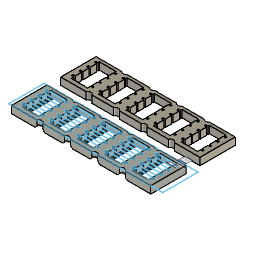
2025_11_30_Stock20Pico2W v6 (Autodesk Fusion 360 design; units mm, degrees)
Autodesk Fusion 360 part; units mm, degrees
note: some values were not read from the file. Set by a fixed rule: which face or edge a step refers to.
sketch "Sketch1" plane through (0, 0, 0) normal (0, 0, 1) x (1, 0, 0)
  line L0 (71.5, 36) -> (-71.5, 36)
  line L1 (-71.5, 36) -> (-71.5, -36)
  line L2 (-71.5, -36) -> (71.5, -36)
  line L3 (71.5, -36) -> (71.5, 36)
  line L4 (71.5, 36) -> (-71.5, -36) construction
  line L5 (-71.5, 36) -> (71.5, -36) construction
  line L6 (71.5, -36) -> (96.5, -36)
  line L7 (96.5, -36) -> (96.5, -14)
  line L8 (96.5, -14) -> (71.5, -14)
  line L9 (71.5, -14) -> (71.5, -36)
  line L10 (71.5, 36) -> (96.5, 36)
  line L11 (96.5, 36) -> (96.5, 14)
  line L12 (96.5, 14) -> (71.5, 14)
  line L13 (71.5, 14) -> (71.5, 36)
  line L14 (71.5, 14) -> (96.5, 14)
  line L15 (96.5, 14) -> (96.5, -14)
  line L16 (96.5, -14) -> (71.5, -14)
  line L17 (71.5, -14) -> (71.5, 14)
  dimension "d1" = 143
  dimension "d2" = 72
  dimension "d5" = 25
  dimension "d6" = 22
  dimension "d7" = 22
  constraint horizontal L0
  constraint perpendicular L0 L1
  constraint parallel L0 L2
  constraint parallel L1 L3
  constraint coincident L4 origin
  constraint coincident L5 origin
  constraint horizontal L6
  constraint vertical L7
  constraint horizontal L8
  constraint vertical L9
  constraint horizontal L10
  constraint vertical L11
  constraint horizontal L12
  constraint vertical L13
  constraint horizontal L14
  constraint vertical L15
  constraint horizontal L16
  constraint vertical L17
  measures "d1" distance of L1.end L2.end
  measures "d2" distance of L0.end L1.end
  measures "d5" distance of L2.end L6.end
  measures "d6" distance of L2.end L8.end
  measures "d7" distance of L0.start L12.end
extrude "Extrude1" add sketch "Sketch1" along normal blind 65 contours L0 L1 L2 L3 L9 L13 L17 makes body 1
sketch "Sketch2" plane through (0, 0, 0) normal (0, 0, 1) x (1, 0, 0)
  line L0 (67.3908, -47.7259) -> (44.3908, -47.7259)
  line L1 (44.3908, -47.7259) -> (44.3908, -49.2259)
  line L2 (44.3908, -49.2259) -> (67.3908, -49.2259)
  line L3 (67.3908, -49.2259) -> (67.3908, -47.7259)
  line L4 (64.8908, -52.2259) -> (46.8908, -52.2259)
  line L5 (46.8908, -52.2259) -> (46.8908, -47.7259)
  line L6 (64.8908, -47.7259) -> (64.8908, -52.2259)
  line L7 (64.8908, -52.2259) -> (51.3908, -47.7259) construction
  line L8 (46.8908, -52.2259) -> (60.3908, -47.7259) construction
  point P0 (55.8908, -49.2259)
  dimension "d8" = 23
  dimension "d9" = 1.5
  constraint horizontal L0
  constraint vertical L1
  constraint horizontal L2
  constraint vertical L3
  constraint horizontal L4
  constraint perpendicular L4 L5
  constraint parallel L5 L6
  constraint coincident L7 P0
  constraint coincident L8 P0
  constraint midpoint L2 P0
  constraint coincident L0 L6.start
  constraint coincident L0 L5.end
  constraint coincident L0 L7.end
  constraint coincident L0 L8.end
  measures "d8" distance of L0.start L0.end
  measures "d9" distance of L0.start L2.end
extrude "Extrude2" add sketch "Sketch2" along normal blind 53 separate body makes body 2
move_body "Move1" bodies 2 to x (1, 0, 0) y (0, 1, 0) z (0, 0, 1) at (-116.4135, 7.0499, 0)
pattern_linear "R-Pattern1" count 5 spacing 30 along (1, 0, 0) count 4 spacing 8.3333 along (0, -1, 0) of bodies 2 makes body 3 at (-33.5227, -40.676, 35.3333) makes body 4 at (-3.5227, -40.676, 35.3333) makes body 5 at (26.4773, -40.676, 35.3333) makes body 6 at (56.4773, -40.676, 35.3333) makes body 7 at (-63.5227, -49.0094, 35.3333) makes body 8 at (-33.5227, -49.0094, 35.3333) makes body 9 at (-3.5227, -49.0094, 35.3333) makes body 10 at (26.4773, -49.0094, 35.3333) makes body 11 at (56.4773, -49.0094, 35.3333) makes body 12 at (-63.5227, -57.3427, 35.3333) makes body 13 at (-33.5227, -57.3427, 35.3333) makes body 14 at (-3.5227, -57.3427, 35.3333) makes body 15 at (26.4773, -57.3427, 35.3333) makes body 16 at (56.4773, -57.3427, 35.3333) makes body 17 at (-63.5227, -65.676, 35.3333) makes body 18 at (-33.5227, -65.676, 35.3333) makes body 19 at (-3.5227, -65.676, 35.3333) makes body 20 at (26.4773, -65.676, 35.3333) makes body 21 at (56.4773, -65.676, 35.3333)
sketch "Sketch3" plane through (0, 0, 0) normal (0, 0, 1) x (1, 0, 0)
  line L0 (-71.5, -36) -> (96.5, -36)
  line L1 (96.5, -36) -> (96.5, -74.6244)
  line L2 (96.5, -74.6244) -> (-71.5, -74.6244)
  line L3 (-71.5, -74.6244) -> (-71.5, -36)
  point P0 (-71.5, -36)
  constraint horizontal L0
  constraint vertical L1
  constraint horizontal L2
  constraint vertical L3
  constraint coincident P0 L0.start
move_body "Move2" bodies 11 2 18 9 3 15 19 8 10 13 5 6 14 17 16 20 4 21 7 12 to x (1, 0, 0) y (0, 1, 0) z (0, 0, 1) at (5, 0, 0)
move_body "Move3" bodies 3 4 10 21 2 13 17 12 15 7 16 18 5 9 19 6 11 8 14 20 to x (1, 0, 0) y (0, 1, 0) z (0, 0, 1) at (3, 0, 0)
move_body "Move4" bodies 7 18 4 10 19 14 11 5 8 2 15 6 17 3 12 13 21 20 9 16 to x (1, 0, 0) y (0, 1, 0) z (0, 0, 1) at (0, 0, 1.5)
extrude "Extrude3" add sketch "Sketch3" along normal blind 8 separate body makes body 22
combine "Combine1" operation cut target body 22 tool bodies 21 16 11 6 20 10 5 15 9 4 14 19 13 8 3 18 2 7 12 17
sketch "Sketch6" plane through (0, 0, 8) normal (0, 0, 1) x (-1, 0, 0)
  line L0 (43.5227, 67.176) -> (43.5227, 70.176)
  line L1 (43.5227, 70.176) -> (61.5227, 70.176)
  line L2 (61.5227, 70.176) -> (61.5227, 67.176)
  line L3 (61.5227, 67.176) -> (64.0227, 67.176)
  line L4 (64.0227, 67.176) -> (64.0227, 65.676)
  line L5 (64.0227, 65.676) -> (41.0227, 65.676)
  line L6 (41.0227, 65.676) -> (41.0227, 67.176)
  line L7 (41.0227, 67.176) -> (43.5227, 67.176)
  line L8 (43.5227, 58.8427) -> (43.5227, 61.8427)
  line L9 (43.5227, 61.8427) -> (61.5227, 61.8427)
  line L10 (61.5227, 61.8427) -> (61.5227, 58.8427)
  line L11 (61.5227, 58.8427) -> (64.0227, 58.8427)
  line L12 (64.0227, 58.8427) -> (64.0227, 57.3427)
  line L13 (64.0227, 57.3427) -> (41.0227, 57.3427)
  line L14 (41.0227, 57.3427) -> (41.0227, 58.8427)
  line L15 (41.0227, 58.8427) -> (43.5227, 58.8427)
  line L16 (43.5227, 50.5094) -> (43.5227, 53.5094)
  line L17 (43.5227, 53.5094) -> (61.5227, 53.5094)
  line L18 (61.5227, 53.5094) -> (61.5227, 50.5094)
  line L19 (61.5227, 50.5094) -> (64.0227, 50.5094)
  line L20 (64.0227, 50.5094) -> (64.0227, 49.0094)
  line L21 (64.0227, 49.0094) -> (41.0227, 49.0094)
  line L22 (41.0227, 49.0094) -> (41.0227, 50.5094)
  line L23 (41.0227, 50.5094) -> (43.5227, 50.5094)
  line L24 (43.5227, 42.176) -> (43.5227, 45.176)
  line L25 (43.5227, 45.176) -> (61.5227, 45.176)
  line L26 (61.5227, 45.176) -> (61.5227, 42.176)
  line L27 (61.5227, 42.176) -> (64.0227, 42.176)
  line L28 (64.0227, 42.176) -> (64.0227, 40.676)
  line L29 (64.0227, 40.676) -> (41.0227, 40.676)
  line L30 (41.0227, 40.676) -> (41.0227, 42.176)
  line L31 (41.0227, 42.176) -> (43.5227, 42.176)
  line L32 (13.5227, 67.176) -> (13.5227, 70.176)
  line L33 (13.5227, 70.176) -> (31.5227, 70.176)
  line L34 (31.5227, 70.176) -> (31.5227, 67.176)
  line L35 (31.5227, 67.176) -> (34.0227, 67.176)
  line L36 (34.0227, 67.176) -> (34.0227, 65.676)
  line L37 (34.0227, 65.676) -> (11.0227, 65.676)
  line L38 (11.0227, 65.676) -> (11.0227, 67.176)
  line L39 (11.0227, 67.176) -> (13.5227, 67.176)
  line L40 (13.5227, 42.176) -> (13.5227, 45.176)
  line L41 (13.5227, 45.176) -> (31.5227, 45.176)
  line L42 (31.5227, 45.176) -> (31.5227, 42.176)
  line L43 (31.5227, 42.176) -> (34.0227, 42.176)
  line L44 (34.0227, 42.176) -> (34.0227, 40.676)
  line L45 (34.0227, 40.676) -> (11.0227, 40.676)
  line L46 (11.0227, 40.676) -> (11.0227, 42.176)
  line L47 (11.0227, 42.176) -> (13.5227, 42.176)
  line L48 (13.5227, 50.5094) -> (13.5227, 53.5094)
  line L49 (13.5227, 53.5094) -> (31.5227, 53.5094)
  line L50 (31.5227, 53.5094) -> (31.5227, 50.5094)
  line L51 (31.5227, 50.5094) -> (34.0227, 50.5094)
  line L52 (34.0227, 50.5094) -> (34.0227, 49.0094)
  line L53 (34.0227, 49.0094) -> (11.0227, 49.0094)
  line L54 (11.0227, 49.0094) -> (11.0227, 50.5094)
  line L55 (11.0227, 50.5094) -> (13.5227, 50.5094)
  line L56 (13.5227, 58.8427) -> (13.5227, 61.8427)
  line L57 (13.5227, 61.8427) -> (31.5227, 61.8427)
  line L58 (31.5227, 61.8427) -> (31.5227, 58.8427)
  line L59 (31.5227, 58.8427) -> (34.0227, 58.8427)
  line L60 (34.0227, 58.8427) -> (34.0227, 57.3427)
  line L61 (34.0227, 57.3427) -> (11.0227, 57.3427)
  line L62 (11.0227, 57.3427) -> (11.0227, 58.8427)
  line L63 (11.0227, 58.8427) -> (13.5227, 58.8427)
  line L64 (-16.4773, 67.176) -> (-16.4773, 70.176)
  line L65 (-16.4773, 70.176) -> (1.5227, 70.176)
  line L66 (1.5227, 70.176) -> (1.5227, 67.176)
  line L67 (1.5227, 67.176) -> (4.0227, 67.176)
  line L68 (4.0227, 67.176) -> (4.0227, 65.676)
  line L69 (4.0227, 65.676) -> (-18.9773, 65.676)
  line L70 (-18.9773, 65.676) -> (-18.9773, 67.176)
  line L71 (-18.9773, 67.176) -> (-16.4773, 67.176)
  line L72 (-16.4773, 58.8427) -> (-16.4773, 61.8427)
  line L73 (-16.4773, 61.8427) -> (1.5227, 61.8427)
  line L74 (1.5227, 61.8427) -> (1.5227, 58.8427)
  line L75 (1.5227, 58.8427) -> (4.0227, 58.8427)
  line L76 (4.0227, 58.8427) -> (4.0227, 57.3427)
  line L77 (4.0227, 57.3427) -> (-18.9773, 57.3427)
  line L78 (-18.9773, 57.3427) -> (-18.9773, 58.8427)
  line L79 (-18.9773, 58.8427) -> (-16.4773, 58.8427)
  line L80 (-16.4773, 42.176) -> (-16.4773, 45.176)
  line L81 (-16.4773, 45.176) -> (1.5227, 45.176)
  line L82 (1.5227, 45.176) -> (1.5227, 42.176)
  line L83 (1.5227, 42.176) -> (4.0227, 42.176)
  line L84 (4.0227, 42.176) -> (4.0227, 40.676)
  line L85 (4.0227, 40.676) -> (-18.9773, 40.676)
  line L86 (-18.9773, 40.676) -> (-18.9773, 42.176)
  line L87 (-18.9773, 42.176) -> (-16.4773, 42.176)
  line L88 (-16.4773, 50.5094) -> (-16.4773, 53.5094)
  line L89 (-16.4773, 53.5094) -> (1.5227, 53.5094)
  line L90 (1.5227, 53.5094) -> (1.5227, 50.5094)
  line L91 (1.5227, 50.5094) -> (4.0227, 50.5094)
  line L92 (4.0227, 50.5094) -> (4.0227, 49.0094)
  line L93 (4.0227, 49.0094) -> (-18.9773, 49.0094)
  line L94 (-18.9773, 49.0094) -> (-18.9773, 50.5094)
  line L95 (-18.9773, 50.5094) -> (-16.4773, 50.5094)
  line L96 (-46.4773, 58.8427) -> (-46.4773, 61.8427)
  line L97 (-46.4773, 61.8427) -> (-28.4773, 61.8427)
  line L98 (-28.4773, 61.8427) -> (-28.4773, 58.8427)
  line L99 (-28.4773, 58.8427) -> (-25.9773, 58.8427)
  line L100 (-25.9773, 58.8427) -> (-25.9773, 57.3427)
  line L101 (-25.9773, 57.3427) -> (-48.9773, 57.3427)
  line L102 (-48.9773, 57.3427) -> (-48.9773, 58.8427)
  line L103 (-48.9773, 58.8427) -> (-46.4773, 58.8427)
  line L104 (-46.4773, 42.176) -> (-46.4773, 45.176)
  line L105 (-46.4773, 45.176) -> (-28.4773, 45.176)
  line L106 (-28.4773, 45.176) -> (-28.4773, 42.176)
  line L107 (-28.4773, 42.176) -> (-25.9773, 42.176)
  line L108 (-25.9773, 42.176) -> (-25.9773, 40.676)
  line L109 (-25.9773, 40.676) -> (-48.9773, 40.676)
  line L110 (-48.9773, 40.676) -> (-48.9773, 42.176)
  line L111 (-48.9773, 42.176) -> (-46.4773, 42.176)
  line L112 (-46.4773, 50.5094) -> (-46.4773, 53.5094)
  line L113 (-46.4773, 53.5094) -> (-28.4773, 53.5094)
  line L114 (-28.4773, 53.5094) -> (-28.4773, 50.5094)
  line L115 (-28.4773, 50.5094) -> (-25.9773, 50.5094)
  line L116 (-25.9773, 50.5094) -> (-25.9773, 49.0094)
  line L117 (-25.9773, 49.0094) -> (-48.9773, 49.0094)
  line L118 (-48.9773, 49.0094) -> (-48.9773, 50.5094)
  line L119 (-48.9773, 50.5094) -> (-46.4773, 50.5094)
  line L120 (-46.4773, 67.176) -> (-46.4773, 70.176)
  line L121 (-46.4773, 70.176) -> (-28.4773, 70.176)
  line L122 (-28.4773, 70.176) -> (-28.4773, 67.176)
  line L123 (-28.4773, 67.176) -> (-25.9773, 67.176)
  line L124 (-25.9773, 67.176) -> (-25.9773, 65.676)
  line L125 (-25.9773, 65.676) -> (-48.9773, 65.676)
  line L126 (-48.9773, 65.676) -> (-48.9773, 67.176)
  line L127 (-48.9773, 67.176) -> (-46.4773, 67.176)
  line L128 (-76.4773, 42.176) -> (-76.4773, 45.176)
  line L129 (-76.4773, 45.176) -> (-58.4773, 45.176)
  line L130 (-58.4773, 45.176) -> (-58.4773, 42.176)
  line L131 (-58.4773, 42.176) -> (-55.9773, 42.176)
  line L132 (-55.9773, 42.176) -> (-55.9773, 40.676)
  line L133 (-55.9773, 40.676) -> (-78.9773, 40.676)
  line L134 (-78.9773, 40.676) -> (-78.9773, 42.176)
  line L135 (-78.9773, 42.176) -> (-76.4773, 42.176)
  line L136 (-76.4773, 50.5094) -> (-76.4773, 53.5094)
  line L137 (-76.4773, 53.5094) -> (-58.4773, 53.5094)
  line L138 (-58.4773, 53.5094) -> (-58.4773, 50.5094)
  line L139 (-58.4773, 50.5094) -> (-55.9773, 50.5094)
  line L140 (-55.9773, 50.5094) -> (-55.9773, 49.0094)
  line L141 (-55.9773, 49.0094) -> (-78.9773, 49.0094)
  line L142 (-78.9773, 49.0094) -> (-78.9773, 50.5094)
  line L143 (-78.9773, 50.5094) -> (-76.4773, 50.5094)
  line L144 (-76.4773, 58.8427) -> (-76.4773, 61.8427)
  line L145 (-76.4773, 61.8427) -> (-58.4773, 61.8427)
  line L146 (-58.4773, 61.8427) -> (-58.4773, 58.8427)
  line L147 (-58.4773, 58.8427) -> (-55.9773, 58.8427)
  line L148 (-55.9773, 58.8427) -> (-55.9773, 57.3427)
  line L149 (-55.9773, 57.3427) -> (-78.9773, 57.3427)
  line L150 (-78.9773, 57.3427) -> (-78.9773, 58.8427)
  line L151 (-78.9773, 58.8427) -> (-76.4773, 58.8427)
  line L152 (-76.4773, 67.176) -> (-76.4773, 70.176)
  line L153 (-76.4773, 70.176) -> (-58.4773, 70.176)
  line L154 (-58.4773, 70.176) -> (-58.4773, 67.176)
  line L155 (-58.4773, 67.176) -> (-55.9773, 67.176)
  line L156 (-55.9773, 67.176) -> (-55.9773, 65.676)
  line L157 (-55.9773, 65.676) -> (-78.9773, 65.676)
  line L158 (-78.9773, 65.676) -> (-78.9773, 67.176)
  line L159 (-78.9773, 67.176) -> (-76.4773, 67.176)
  line L160 (71.5, 74.6244) -> (-96.5, 74.6244)
  line L161 (-96.5, 74.6244) -> (-96.5, 36)
  line L162 (-96.5, 36) -> (71.5, 36)
  line L163 (71.5, 36) -> (71.5, 74.6244)
  line L164 (-96.5, 74.6244) -> (-96.5, 36)
  line L165 (34.0227, 40.676) -> (11.0227, 40.676)
  line L166 (34.0227, 49.0094) -> (11.0227, 49.0094)
  line L167 (-46.4773, 70.176) -> (-28.4773, 70.176)
  line L168 (-25.9773, 49.0094) -> (-48.9773, 49.0094)
  line L169 (-96.5, 36) -> (71.5, 36)
  line L170 (-25.9773, 65.676) -> (-48.9773, 65.676)
  line L171 (34.0227, 57.3427) -> (11.0227, 57.3427)
  line L172 (71.5, 74.6244) -> (-96.5, 74.6244)
  line L173 (4.0227, 50.5094) -> (4.0227, 49.0094)
  line L174 (11.0227, 58.8427) -> (13.5227, 58.8427)
  line L175 (-25.9773, 42.176) -> (-25.9773, 40.676)
  line L176 (-76.4773, 58.8427) -> (-76.4773, 61.8427)
  line L177 (31.5227, 61.8427) -> (31.5227, 58.8427)
  line L178 (-58.4773, 45.176) -> (-58.4773, 42.176)
  line L179 (61.5227, 45.176) -> (61.5227, 42.176)
  line L180 (43.5227, 50.5094) -> (43.5227, 53.5094)
  line L181 (61.5227, 42.176) -> (64.0227, 42.176)
  line L182 (11.0227, 57.3427) -> (11.0227, 58.8427)
  line L183 (1.5227, 45.176) -> (1.5227, 42.176)
  line L184 (-76.4773, 61.8427) -> (-58.4773, 61.8427)
  line L185 (-48.9773, 49.0094) -> (-48.9773, 50.5094)
  line L186 (-48.9773, 57.3427) -> (-48.9773, 58.8427)
  line L187 (-78.9773, 67.176) -> (-76.4773, 67.176)
  line L188 (64.0227, 40.676) -> (41.0227, 40.676)
  line L189 (-55.9773, 49.0094) -> (-78.9773, 49.0094)
  line L190 (-25.9773, 67.176) -> (-25.9773, 65.676)
  line L191 (-46.4773, 58.8427) -> (-46.4773, 61.8427)
  line L192 (43.5227, 61.8427) -> (61.5227, 61.8427)
  line L193 (4.0227, 42.176) -> (4.0227, 40.676)
  line L194 (64.0227, 57.3427) -> (41.0227, 57.3427)
  line L195 (-78.9773, 65.676) -> (-78.9773, 67.176)
  line L196 (-28.4773, 58.8427) -> (-25.9773, 58.8427)
  line L197 (11.0227, 42.176) -> (13.5227, 42.176)
  line L198 (-76.4773, 42.176) -> (-76.4773, 45.176)
  line L199 (34.0227, 58.8427) -> (34.0227, 57.3427)
  line L200 (34.0227, 50.5094) -> (34.0227, 49.0094)
  line L201 (13.5227, 45.176) -> (31.5227, 45.176)
  line L202 (-28.4773, 70.176) -> (-28.4773, 67.176)
  line L203 (-28.4773, 50.5094) -> (-25.9773, 50.5094)
  line L204 (-25.9773, 58.8427) -> (-25.9773, 57.3427)
  line L205 (-48.9773, 50.5094) -> (-46.4773, 50.5094)
  line L206 (-18.9773, 57.3427) -> (-18.9773, 58.8427)
  line L207 (-76.4773, 45.176) -> (-58.4773, 45.176)
  line L208 (64.0227, 42.176) -> (64.0227, 40.676)
  line L209 (31.5227, 58.8427) -> (34.0227, 58.8427)
  line L210 (-28.4773, 42.176) -> (-25.9773, 42.176)
  line L211 (31.5227, 50.5094) -> (34.0227, 50.5094)
  line L212 (1.5227, 50.5094) -> (4.0227, 50.5094)
  line L213 (-16.4773, 45.176) -> (1.5227, 45.176)
  line L214 (-48.9773, 58.8427) -> (-46.4773, 58.8427)
  line L215 (-48.9773, 67.176) -> (-46.4773, 67.176)
  line L216 (64.0227, 49.0094) -> (41.0227, 49.0094)
  line L217 (-28.4773, 67.176) -> (-25.9773, 67.176)
  line L218 (-48.9773, 65.676) -> (-48.9773, 67.176)
  line L219 (43.5227, 45.176) -> (61.5227, 45.176)
  line L220 (-28.4773, 61.8427) -> (-28.4773, 58.8427)
  line L221 (64.0227, 65.676) -> (41.0227, 65.676)
  line L222 (-25.9773, 50.5094) -> (-25.9773, 49.0094)
  line L223 (11.0227, 40.676) -> (11.0227, 42.176)
  line L224 (4.0227, 49.0094) -> (-18.9773, 49.0094)
  line L225 (13.5227, 42.176) -> (13.5227, 45.176)
  line L226 (43.5227, 53.5094) -> (61.5227, 53.5094)
  line L227 (-25.9773, 40.676) -> (-48.9773, 40.676)
  line L228 (-46.4773, 61.8427) -> (-28.4773, 61.8427)
  line L229 (-78.9773, 49.0094) -> (-78.9773, 50.5094)
  line L230 (-46.4773, 45.176) -> (-28.4773, 45.176)
  line L231 (4.0227, 40.676) -> (-18.9773, 40.676)
  line L232 (71.5, 36) -> (71.5, 74.6244)
  line L233 (-78.9773, 50.5094) -> (-76.4773, 50.5094)
  line L234 (-46.4773, 53.5094) -> (-28.4773, 53.5094)
  line L235 (-25.9773, 57.3427) -> (-48.9773, 57.3427)
  line L236 (34.0227, 65.676) -> (11.0227, 65.676)
  line L237 (-18.9773, 58.8427) -> (-16.4773, 58.8427)
  line L238 (-46.4773, 67.176) -> (-46.4773, 70.176)
  line L239 (-55.9773, 65.676) -> (-78.9773, 65.676)
  line L240 (43.5227, 70.176) -> (61.5227, 70.176)
  line L241 (34.0227, 67.176) -> (34.0227, 65.676)
  line L242 (-58.4773, 42.176) -> (-55.9773, 42.176)
  line L243 (31.5227, 53.5094) -> (31.5227, 50.5094)
  line L244 (-28.4773, 53.5094) -> (-28.4773, 50.5094)
  line L245 (13.5227, 61.8427) -> (31.5227, 61.8427)
  line L246 (-18.9773, 50.5094) -> (-16.4773, 50.5094)
  line L247 (-16.4773, 58.8427) -> (-16.4773, 61.8427)
  line L248 (1.5227, 42.176) -> (4.0227, 42.176)
  line L249 (1.5227, 53.5094) -> (1.5227, 50.5094)
  line L250 (-18.9773, 49.0094) -> (-18.9773, 50.5094)
  line L251 (-58.4773, 61.8427) -> (-58.4773, 58.8427)
  line L252 (-55.9773, 42.176) -> (-55.9773, 40.676)
  line L253 (-18.9773, 65.676) -> (-18.9773, 67.176)
  line L254 (-58.4773, 58.8427) -> (-55.9773, 58.8427)
  line L255 (34.0227, 42.176) -> (34.0227, 40.676)
  line L256 (-46.4773, 42.176) -> (-46.4773, 45.176)
  line L257 (-46.4773, 50.5094) -> (-46.4773, 53.5094)
  line L258 (-18.9773, 67.176) -> (-16.4773, 67.176)
  line L259 (-16.4773, 53.5094) -> (1.5227, 53.5094)
  line L260 (64.0227, 50.5094) -> (64.0227, 49.0094)
  line L261 (13.5227, 58.8427) -> (13.5227, 61.8427)
  line L262 (31.5227, 67.176) -> (34.0227, 67.176)
  line L263 (4.0227, 58.8427) -> (4.0227, 57.3427)
  line L264 (61.5227, 50.5094) -> (64.0227, 50.5094)
  line L265 (11.0227, 50.5094) -> (13.5227, 50.5094)
  line L266 (-16.4773, 50.5094) -> (-16.4773, 53.5094)
  line L267 (4.0227, 57.3427) -> (-18.9773, 57.3427)
  line L268 (-16.4773, 67.176) -> (-16.4773, 70.176)
  line L269 (-16.4773, 70.176) -> (1.5227, 70.176)
  line L270 (-55.9773, 58.8427) -> (-55.9773, 57.3427)
  line L271 (-48.9773, 42.176) -> (-46.4773, 42.176)
  line L272 (-55.9773, 40.676) -> (-78.9773, 40.676)
  line L273 (31.5227, 42.176) -> (34.0227, 42.176)
  line L274 (61.5227, 53.5094) -> (61.5227, 50.5094)
  line L275 (31.5227, 70.176) -> (31.5227, 67.176)
  line L276 (-28.4773, 45.176) -> (-28.4773, 42.176)
  line L277 (-18.9773, 40.676) -> (-18.9773, 42.176)
  line L278 (-78.9773, 57.3427) -> (-78.9773, 58.8427)
  line L279 (11.0227, 49.0094) -> (11.0227, 50.5094)
  line L280 (-48.9773, 40.676) -> (-48.9773, 42.176)
  line L281 (-55.9773, 67.176) -> (-55.9773, 65.676)
  line L282 (41.0227, 58.8427) -> (43.5227, 58.8427)
  line L283 (31.5227, 45.176) -> (31.5227, 42.176)
  line L284 (41.0227, 57.3427) -> (41.0227, 58.8427)
  line L285 (-18.9773, 42.176) -> (-16.4773, 42.176)
  line L286 (1.5227, 58.8427) -> (4.0227, 58.8427)
  line L287 (-55.9773, 57.3427) -> (-78.9773, 57.3427)
  line L288 (43.5227, 67.176) -> (43.5227, 70.176)
  line L289 (41.0227, 49.0094) -> (41.0227, 50.5094)
  line L290 (-78.9773, 40.676) -> (-78.9773, 42.176)
  line L291 (-55.9773, 50.5094) -> (-55.9773, 49.0094)
  line L292 (1.5227, 61.8427) -> (1.5227, 58.8427)
  line L293 (-78.9773, 42.176) -> (-76.4773, 42.176)
  line L294 (13.5227, 53.5094) -> (31.5227, 53.5094)
  line L295 (41.0227, 42.176) -> (43.5227, 42.176)
  line L296 (-78.9773, 58.8427) -> (-76.4773, 58.8427)
  line L297 (13.5227, 50.5094) -> (13.5227, 53.5094)
  line L298 (43.5227, 58.8427) -> (43.5227, 61.8427)
  line L299 (41.0227, 50.5094) -> (43.5227, 50.5094)
  line L300 (64.0227, 58.8427) -> (64.0227, 57.3427)
  line L301 (-16.4773, 42.176) -> (-16.4773, 45.176)
  line L302 (13.5227, 67.176) -> (13.5227, 70.176)
  line L303 (13.5227, 70.176) -> (31.5227, 70.176)
  line L304 (-76.4773, 53.5094) -> (-58.4773, 53.5094)
  line L305 (11.0227, 65.676) -> (11.0227, 67.176)
  line L306 (41.0227, 40.676) -> (41.0227, 42.176)
  line L307 (-76.4773, 67.176) -> (-76.4773, 70.176)
  line L308 (1.5227, 70.176) -> (1.5227, 67.176)
  line L309 (41.0227, 67.176) -> (43.5227, 67.176)
  line L310 (11.0227, 67.176) -> (13.5227, 67.176)
  line L311 (61.5227, 58.8427) -> (64.0227, 58.8427)
  line L312 (-76.4773, 50.5094) -> (-76.4773, 53.5094)
  line L313 (41.0227, 65.676) -> (41.0227, 67.176)
  line L314 (61.5227, 61.8427) -> (61.5227, 58.8427)
  line L315 (-58.4773, 50.5094) -> (-55.9773, 50.5094)
  line L316 (-58.4773, 67.176) -> (-55.9773, 67.176)
  line L317 (43.5227, 42.176) -> (43.5227, 45.176)
  line L318 (-58.4773, 70.176) -> (-58.4773, 67.176)
  line L319 (-76.4773, 70.176) -> (-58.4773, 70.176)
  line L320 (1.5227, 67.176) -> (4.0227, 67.176)
  line L321 (61.5227, 70.176) -> (61.5227, 67.176)
  line L322 (64.0227, 67.176) -> (64.0227, 65.676)
  line L323 (-58.4773, 53.5094) -> (-58.4773, 50.5094)
  line L324 (4.0227, 67.176) -> (4.0227, 65.676)
  line L325 (4.0227, 65.676) -> (-18.9773, 65.676)
  line L326 (-16.4773, 61.8427) -> (1.5227, 61.8427)
  line L327 (61.5227, 67.176) -> (64.0227, 67.176)
extrude "Extrude9" cut 5 faces at (-49.5227, -45.176, 3.6667) (-19.5227, -45.176, 3.6667) (10.4773, -45.176, 3.6667) (40.4773, -45.176, 3.6667) (70.4773, -45.176, 3.6667) along direction (0, 1, 0) blind 6 on bodies 22 bodies 22
extrude "Extrude4" cut 5 faces at (-49.5227, -45.176, 3.6667) (-19.5227, -45.176, 3.6667) (10.4773, -45.176, 3.6667) (40.4773, -45.176, 3.6667) (70.4773, -45.176, 3.6667) along direction (0, -1, 0) blind 25 on bodies 22 bodies 22
extrude "Extrude5" cut 1 faces at (-71.5, -61.7496, 5.3333) along direction (1, 0, 0) blind 3 on bodies 22 bodies 22
extrude "Extrude6" cut 1 faces at (96.5, -48.8748, 5.3333) along direction (-1, 0, 0) blind 13 on bodies 22 bodies 22
sketch "Sketch4" plane through (0, 0, 1.5) normal (0, 0, 1) x (-1, 0, 0)
  line L0 (61.5227, 65.676) -> (64.0227, 65.676)
  line L1 (64.0227, 65.676) -> (64.0227, 67.176)
  line L2 (64.0227, 67.176) -> (61.5227, 67.176)
  line L3 (61.5227, 67.176) -> (61.5227, 70.176)
  line L4 (61.5227, 70.176) -> (43.5227, 70.176)
  line L5 (43.5227, 70.176) -> (43.5227, 67.176)
  line L6 (43.5227, 67.176) -> (41.0227, 67.176)
  line L7 (41.0227, 67.176) -> (41.0227, 65.676)
  line L8 (41.0227, 65.676) -> (43.5227, 65.676)
  line L9 (43.5227, 65.676) -> (43.5227, 58.8427)
  line L10 (43.5227, 58.8427) -> (41.0227, 58.8427)
  line L11 (41.0227, 58.8427) -> (41.0227, 57.3427)
  line L12 (41.0227, 57.3427) -> (43.5227, 57.3427)
  line L13 (43.5227, 57.3427) -> (43.5227, 50.5094)
  line L14 (43.5227, 50.5094) -> (41.0227, 50.5094)
  line L15 (41.0227, 50.5094) -> (41.0227, 49.0094)
  line L16 (41.0227, 49.0094) -> (43.5227, 49.0094)
  line L17 (43.5227, 49.0094) -> (43.5227, 42.176)
  line L18 (43.5227, 42.176) -> (41.0227, 42.176)
  line L19 (41.0227, 42.176) -> (41.0227, 40.676)
  line L20 (41.0227, 40.676) -> (43.5227, 40.676)
  line L21 (64.0227, 40.676) -> (64.0227, 42.176)
  line L22 (64.0227, 42.176) -> (61.5227, 42.176)
  line L23 (61.5227, 42.176) -> (61.5227, 49.0094)
  line L24 (61.5227, 49.0094) -> (64.0227, 49.0094)
  line L25 (64.0227, 49.0094) -> (64.0227, 50.5094)
  line L26 (64.0227, 50.5094) -> (61.5227, 50.5094)
  line L27 (61.5227, 50.5094) -> (61.5227, 57.3427)
  line L28 (61.5227, 57.3427) -> (64.0227, 57.3427)
  line L29 (64.0227, 57.3427) -> (64.0227, 58.8427)
  line L30 (64.0227, 58.8427) -> (61.5227, 58.8427)
  line L31 (61.5227, 58.8427) -> (61.5227, 65.676)
  line L32 (59.7325, 40.676) -> (45.4594, 40.676)
  line L33 (45.4594, 40.676) -> (45.4594, 70.176)
  line L34 (45.4594, 70.176) -> (59.7325, 70.176)
  line L35 (59.7325, 70.176) -> (59.7325, 40.676)
  line L36 (29.7325, 70.176) -> (29.7325, 40.676)
  line L37 (29.7325, 40.676) -> (15.4594, 40.676)
  line L38 (15.4594, 40.676) -> (15.4594, 70.176)
  line L39 (15.4594, 70.176) -> (29.7325, 70.176)
  line L40 (-0.2675, 70.176) -> (-0.2675, 40.676)
  line L41 (-0.2675, 40.676) -> (-14.5406, 40.676)
  line L42 (-14.5406, 40.676) -> (-14.5406, 70.176)
  line L43 (-14.5406, 70.176) -> (-0.2675, 70.176)
  line L44 (-30.2675, 70.176) -> (-30.2675, 40.676)
  line L45 (-30.2675, 40.676) -> (-44.5406, 40.676)
  line L46 (-44.5406, 40.676) -> (-44.5406, 70.176)
  line L47 (-44.5406, 70.176) -> (-30.2675, 70.176)
  line L48 (-60.2675, 70.176) -> (-60.2675, 40.676)
  line L49 (-60.2675, 40.676) -> (-74.5406, 40.676)
  line L50 (-74.5406, 40.676) -> (-74.5406, 70.176)
  line L51 (-74.5406, 70.176) -> (-60.2675, 70.176)
  line L52 (43.5227, 40.676) -> (43.5227, 39.176)
  line L53 (43.5227, 39.176) -> (61.5227, 39.176)
  line L54 (61.5227, 39.176) -> (61.5227, 40.676)
  line L55 (61.5227, 40.676) -> (64.0227, 40.676)
  dimension "d28" = -120
  dimension "d29" = 0
  constraint horizontal L32
  constraint vertical L33
  constraint horizontal L34
  constraint vertical L35
  constraint coincident L4 L33.end
  constraint coincident L20 L32.start
extrude "Extrude7" cut sketch "Sketch4" against normal blind 10 contours L4 L32 L33 L34 L35 | L36 L37 L38 L39 | L40 L41 L42 L43 | L44 L45 L46 L47 | L48 L49 L50 L51 bodies 22
sketch "Sketch5" plane through (0, 0, 0) normal (0, 0, 1) x (1, 0, 0)
  circle A0 centre (-37.5405, -33.9429) radius 3.492
  line L0 (83.5, -36) -> (-68.5, -36)
  line L1 (-41.0227, -40.676) -> (-34.0227, -40.676)
  line L2 (-34.0227, -40.676) -> (-37.5227, -40.676)
  line L3 (-37.5405, -33.9429) -> (-37.5227, -40.676)
  line L4 (-37.5227, -40.676) -> (-37.5405, -83.8674)
  circle A1 centre (-37.5316, -76.0465) radius 3.492
  circle A2 centre (-7.5405, -33.9429) radius 3.492
  circle A3 centre (-7.5316, -76.0465) radius 3.492
  circle A4 centre (22.4595, -33.9429) radius 3.492
  circle A5 centre (22.4684, -76.0465) radius 3.492
  circle A6 centre (52.4595, -33.9429) radius 3.492
  circle A7 centre (52.4684, -76.0465) radius 3.492
  point P0 (-41.0227, -40.676)
  point P1 (-34.0227, -40.676)
  dimension "d34" = 90
  dimension "d35" = 0
  constraint coincident P0 L1.start
  constraint midpoint L1 L2.end
  constraint coincident A0.centre L3.start
extrude "Extrude8" cut sketch "Sketch5" along normal blind 25 bodies 22
fillet "Fillet1" radius 3 8 edges at (52.4684, -72.5544, 0) (22.4684, -72.5544, 0) (-7.5316, -72.5544, 0) (-37.5316, -72.5544, 0) (52.4595, -37.4349, 0) (22.4595, -37.4349, 0) (-7.5405, -37.4349, 0) (-37.5405, -37.4349, 0) on bodies 22
extrude "Extrude10" cut 5 faces at (-54.9748, -40.676, 1) (-24.9748, -40.676, 1) (5.0252, -40.676, 1) (35.0252, -40.676, 1) (65.0252, -40.676, 1) along direction (0, 1, 0) blind 1.5 on bodies 22 bodies 22
fillet "Fillet2" radius 2 10 edges at (-52.596, -39.176, 0) (-22.596, -39.176, 0) (7.404, -39.176, 0) (37.404, -39.176, 0) (67.404, -39.176, 0) (67.404, -70.176, 0) (37.404, -70.176, 0) (7.404, -70.176, 0) (-22.596, -70.176, 0) (-52.596, -70.176, 0) on bodies 22
extrude "Extrude11" add 1 faces at (81.9924, -55.989, 8) along direction (0, 0, 1) blind 8 separate body on bodies 22 makes body 23
move_body "Move5" bodies 23 to x (1, 0, 0) y (0, 1, 0) z (0, 0, 1) at (0, 38.6244, -8)
move_body "Move6" bodies 23 to x (1, 0, 0) y (0, 1, 0) z (0, 0, 1) at (0, 15, 0)
hidden bodies 1
named bodies: "Sticj20Pico2W"
